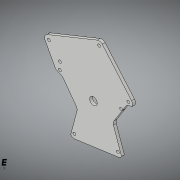
# Autodesk Inventor part: 中間内フレーム
Saved by Autodesk Inventor 2019 (Build 230136000, 136)
## iProperties
Created: 2019-09-17
Part Number: 中間内フレーム
Material: 一般
Document SubType Name: Modeling
Designer: tanjihayato
Density: 1 g/cm^3
Appearance: 既定
Author: tanjihayato
Autodesk Inventor part; units mm, degrees
ref_plane "YZ Plane" through (0, 0, 0) normal (1, 0, 0) x (0, 1, 0)
ref_plane "XZ Plane" through (0, 0, 0) normal (0, 1, 0) x (-1, 0, 0)
ref_plane "XY Plane" through (0, 0, 0) normal (0, 0, 1) x (1, 0, 0)
sketch "スケッチ3" plane through (0, 0, 0) normal (0, 0, 1) x (1, 0, 0)
  circle A0 centre (0, 0) radius 20.55 construction
  circle A1 centre (-21.6908, -16.4118) radius 19.1 construction
  circle A2 centre (25.3202, -9.9362) radius 19.1 construction
  circle A3 centre (-47.0055, 32.2626) radius 1.5
  circle A4 centre (5.9362, 53.5882) radius 1.5
  circle A5 centre (29.1381, 7.2346) radius 1.5
  circle A6 centre (-35.2306, 18.3503) radius 1.5
  circle A7 centre (-21.6908, -16.4118) radius 4.025
  circle A8 centre (25.3202, -9.9362) radius 4.025
  circle A9 centre (0, 0) radius 4
  line L0 (-17.8785, -18.8026) -> (-30.4168, -38.7963) construction
  arc A10 (-17.8785, -18.8026) -> (-19.2493, -12.6317) centre (-21.6908, -16.4118) ccw construction
  line L1 (-19.2493, -12.6317) -> (-39.0737, 0.1727) construction
  line L2 (37.1409, -30.8522) -> (21.8866, -12.8448) construction
  arc A11 (22.3659, -6.5417) -> (21.8866, -12.8448) centre (25.3202, -9.9362) ccw construction
  line L3 (22.3659, -6.5417) -> (40.1678, 8.9519) construction
  line L4 (-21.6908, -16.4118) -> (-99.9742, 13.5882) construction
  line L5 (-105.5257, -16.4118) -> (-21.6908, -16.4118) construction
  line L6 (-21.6908, -16.4118) -> (-101.7113, -41.4118) construction
  line L7 (25.3202, -9.9362) -> (102.5386, -46.4118) construction
  line L8 (110.4743, -16.4118) -> (25.3202, -9.9362) construction
  line L9 (25.3202, -9.9362) -> (108.6869, 8.5882) construction
  line L10 (-18.0583, -13.7557) -> (-31.9879, 5.2949) construction
  line L11 (-17.339, -17.5569) -> (-24.5367, -44.9106) construction
  line L12 (21.5077, -7.5456) -> (34.045, 12.4488) construction
  line L13 (21.0739, -11.4259) -> (31.6059, -41.446) construction
  arc A12 (-24.6176, -40.3201) -> (-19.5065, -44.4166) centre (-20.132, -39.9603) ccw
  circle A13 centre (-20.132, -39.9603) radius 3 construction
  arc A14 (-39.3604, 8.5711) -> (-39.3359, 8.5262) centre (-35.3982, 10.7044) ccw
  circle A15 centre (-35.3982, 10.7044) radius 3 construction
  arc A16 (-31.9879, 5.2949) -> (-33.8465, 6.7744) centre (-35.6204, 2.6388) ccw construction
  circle A17 centre (-41.5152, -3.6073) radius 1.5
  line L14 (-33.8465, 6.7744) -> (-56.066, 16.3055) construction
  line L15 (-41.3386, 0.8892) -> (-72.6317, 2.1181) construction
  circle A18 centre (-35.2306, 18.3503) radius 3 construction
  circle A19 centre (-35.3982, 10.7044) radius 1.5
  circle A20 centre (36.7736, 17.5344) radius 1.5
  arc A21 (40.7942, 15.5132) -> (40.1934, 20.4593) centre (36.7736, 17.5344) ccw
  circle A22 centre (25.6508, -33.5339) radius 1.5
  arc A23 (26.2763, -37.9902) -> (30.1508, -33.5178) centre (25.6508, -33.5339) ccw
  circle A24 centre (36.7736, 17.5344) radius 3 construction
  circle A25 centre (25.6508, -33.5339) radius 3 construction
  arc A26 (36.6836, 14.4025) -> (34.045, 12.4488) centre (37.8575, 10.0583) ccw construction
  line L16 (36.6836, 14.4025) -> (64.1968, 21.8369) construction
  line L17 (43.2599, 10.0553) -> (82.9273, 8.8396) construction
  circle A27 centre (29.1381, 7.2346) radius 3 construction
  circle A28 centre (-21.6908, -16.4118) radius 7.025 construction
  circle A29 centre (25.3202, -9.9362) radius 7.025 construction
  arc A30 (40.8593, 15.6483) -> (30.1508, -33.5178) centre (146.4685, -33.1029) ccw
  arc A31 (-24.6176, -40.3201) -> (-39.3359, 8.5262) centre (-145.1158, -49.988) ccw
  arc A32 (-48.6869, 36.4367) -> (-50.9677, 30.1293) centre (-47.0055, 32.2626) ccw
  arc A33 (9.356, 56.5132) -> (4.2549, 57.7623) centre (5.9362, 53.5882) ccw
  line L18 (-39.3604, 8.5711) -> (-50.9677, 30.1293)
  line L19 (-48.6869, 36.4367) -> (4.2549, 57.7623)
  line L20 (9.356, 56.5132) -> (40.1934, 20.4593)
  line L21 (-19.5065, -44.4166) -> (26.2763, -37.9902)
  circle A34 centre (-20.132, -39.9603) radius 1.5
  dimension "d69" = 8.05
  dimension "d70" = 8.05
  dimension "d71" = 8
  dimension "d72" = 20.968
  dimension "d73" = 20.968
  dimension "d74" = 17.35
  dimension "d75" = 17.35
  dimension "d76" = 16.877
  dimension "d77" = 16.877
  dimension "d78" = 20.936
  dimension "d79" = 20.936
  dimension "d80" = 9
  dimension "d81" = 6
  dimension "d82" = 9
  dimension "d83" = 6
  dimension "d84" = 9
  dimension "d85" = 20.968
  dimension "d86" = 20.968
  dimension "d87" = 6
  dimension "d88" = 3
  dimension "d89" = 3
  dimension "d90" = 9
  dimension "d91" = 3
  dimension "d92" = 9
  dimension "d93" = 6
  dimension "d94" = 6
  dimension "d95" = 9
  dimension "d96" = 16.877
  dimension "d97" = 3
  dimension "d98" = 3
  dimension "d99" = 9
  dimension "d100" = 9
  dimension "d101" = 3
  constraints: 44 end point, 35 centre point, 29 point on circle, 27 tangent, 14 coincident, 2 equal length, 1 point on line
  measures "d69" diameter of A7
  measures "d70" diameter of A8
  measures "d71" diameter of A9
  measures "d72" angle of L5 L4
  measures "d73" angle of L1 L10
  measures "d74" angle of L5 L6
  measures "d75" angle of L0 L11
  measures "d76" angle of L8 L9
  measures "d77" angle of L12 L3
  measures "d78" angle of L8 L7
  measures "d79" angle of L13 L2
  measures "d80" diameter of A12
  measures "d81" diameter of A13
  measures "d82" diameter of A14
  measures "d83" diameter of A15
  measures "d84" diameter of A16
  measures "d86" angle of L15 L14
  measures "d87" diameter of A18
  measures "d88" diameter of A19
  measures "d89" diameter of A20
  measures "d90" diameter of A21
  measures "d91" diameter of A22
  measures "d92" diameter of A23
  measures "d93" diameter of A24
  measures "d94" diameter of A25
  measures "d95" diameter of A26
  measures "d96" angle of L16 L17
  measures "d97" radial gap between concentric circles of A7 A28
  measures "d98" radial gap between concentric circles of A8 A29
  measures "d99" diameter of A32
  measures "d100" diameter of A33
  measures "d101" diameter of A34
extrude "押し出し3" add sketch "スケッチ3" along normal blind 3 contours A31 A14 L18 A32 L19 A33 L20 A21 A30 A23 L21 A12
sketch "スケッチ4" plane through (0, 0, 3) normal (0, 0, 1) x (1, 0, 0)
  line L0 (21.5077, -7.5456) -> (34.045, 12.4488) projected
  line L1 (21.0739, -11.4259) -> (31.6059, -41.446) projected
  arc A0 (36.6836, 14.4025) -> (34.045, 12.4488) centre (37.8575, 10.0583) ccw projected
  line L2 (36.6836, 14.4025) -> (64.1968, 21.8369) projected
  line L3 (-33.8465, 6.7744) -> (-56.066, 16.3055) projected
  arc A1 (-31.9879, 5.2949) -> (-33.8465, 6.7744) centre (-35.6204, 2.6388) ccw projected
  line L4 (-18.0583, -13.7557) -> (-31.9879, 5.2949) projected
  line L5 (-17.339, -17.5569) -> (-24.5367, -44.9106) projected
  circle A2 centre (25.3202, -9.9362) radius 4.025 projected
  circle A3 centre (-21.6908, -16.4118) radius 4.025 projected
  circle A4 centre (0, 0) radius 4 projected
  circle A5 centre (-20.132, -39.9603) radius 1.5 projected
  circle A6 centre (25.6508, -33.5339) radius 1.5 projected
  circle A7 centre (36.7736, 17.5344) radius 1.5 projected
  circle A8 centre (-35.3982, 10.7044) radius 1.5 projected
  circle A9 centre (-35.2306, 18.3503) radius 1.5 projected
  circle A10 centre (29.1381, 7.2346) radius 1.5 projected
  circle A11 centre (5.9362, 53.5882) radius 1.5 projected
  circle A12 centre (-47.0055, 32.2626) radius 1.5 projected
  arc A13 (-24.6176, -40.3201) -> (-19.5065, -44.4166) centre (-20.132, -39.9603) ccw projected
  line L6 (-19.5065, -44.4166) -> (26.2763, -37.9902) projected
  arc A14 (26.2763, -37.9902) -> (30.1508, -33.5178) centre (25.6508, -33.5339) ccw projected
  arc A15 (40.8593, 15.6483) -> (30.1508, -33.5178) centre (146.4685, -33.1029) ccw projected
  arc A16 (40.8593, 15.6483) -> (40.1934, 20.4593) centre (36.7736, 17.5344) ccw projected
  line L7 (40.1934, 20.4593) -> (9.356, 56.5132) projected
  arc A17 (9.356, 56.5132) -> (4.2549, 57.7623) centre (5.9362, 53.5882) ccw projected
  line L8 (4.2549, 57.7623) -> (-48.6869, 36.4367) projected
  arc A18 (-48.6869, 36.4367) -> (-50.9677, 30.1293) centre (-47.0055, 32.2626) ccw projected
  line L9 (-50.9677, 30.1293) -> (-39.3604, 8.5711) projected
  arc A19 (-39.3604, 8.5711) -> (-39.3359, 8.5262) centre (-35.3982, 10.7044) ccw projected
  arc A20 (-24.6176, -40.3201) -> (-39.3359, 8.5262) centre (-145.1158, -49.988) ccw projected
  arc A21 (-17.339, -17.5569) -> (-18.0583, -13.7557) centre (-21.6908, -16.4118) ccw
  arc A22 (21.5077, -7.5456) -> (21.0739, -11.4259) centre (25.3202, -9.9362) ccw
  line L10 (-39.7585, 9.3104) -> (-33.8465, 6.7744)
  line L11 (-17.339, -17.5569) -> (-23.8868, -42.4405)
  arc A23 (40.8593, 15.6483) -> (30.1508, -33.5178) centre (146.4685, -33.1029) ccw projected
  line L12 (40.7974, 15.5141) -> (36.6836, 14.4025)
  line L13 (21.0739, -11.4259) -> (29.592, -35.7057)
  constraints: 8 end point, 7 point on circle, 5 point on line, 2 centre point, 2 coincident, 1 collinear
extrude "押し出し4" cut sketch "スケッチ4" against normal blind 10 contours L0 A10 A0 L2 A15 A14 L1 A22 | L0 A10 | A13 A20 A19 L9 L3 A1 L4 A21 L5 picked at (30.2857, 6.4006)
equation "\"d73\" = d72"
equation "\"d75\" = d74"
equation "\"d77\" = d76"
equation "\"d79\" = d78"
equation "\"d85\" = d72"
equation "\"d86\" = d72"
equation "\"d96\" = d76"
